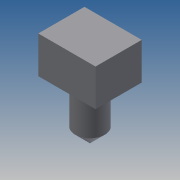
# Autodesk Inventor part: effector
Saved by Autodesk Inventor 2013 (Build 170138000, 138)
## iProperties
Created: 2017-03-06
Part Number: effector
Material: Generic
Document SubType Name: Modeling
Designer: employee
Density: 1 g/cm^3
Author: employee
Autodesk Inventor part; units mm, degrees
ref_plane "YZ Plane" through (0, 0, 0) normal (1, 0, 0) x (0, 1, 0)
ref_plane "XZ Plane" through (0, 0, 0) normal (0, 1, 0) x (-1, 0, 0)
ref_plane "XY Plane" through (0, 0, 0) normal (0, 0, 1) x (1, 0, 0)
sketch "Sketch1" plane through (0, 0, 0) normal (0, 1, 0) x (-1, 0, 0)
  line L0 (0, 0) -> (8, 8)
  line L1 (8, 8) -> (8, 50)
  line L2 (8, 50) -> (0, 50)
  line L3 (0, 50) -> (0, 0)
  dimension "d0" = 50
  dimension "d1" = 8
  dimension "d2" = 135
  constraints: 8 end point, 2 perpendicular, 1 vertical
  measures "d0" distance of L2.end L0.start
  measures "d1" distance between parallel lines of L1 L3
  measures "d2" angle of L3 L0
revolve "Revolution1" add sketch "Sketch1" angle 360 about axis through (0, 0, 50) along (0, 0, -1)
sketch "Sketch2" plane through (0, 0, 50) normal (0, 0, 1) x (1, 0, 0)
  circle A0 centre (0, 0) radius 8 projected
  line L0 (-15.5, -12.5) -> (15.5, -12.5)
  line L1 (15.5, -12.5) -> (15.5, 12.5)
  line L2 (15.5, 12.5) -> (-15.5, 12.5)
  line L3 (-15.5, 12.5) -> (-15.5, -12.5)
  line L4 (-15.5, -12.5) -> (15.5, 12.5) construction
  line L5 (15.5, -12.5) -> (-15.5, 12.5) construction
  dimension "d4" = 31
  dimension "d6" = 25
  constraints: 12 end point, 2 midpoint, 2 parallel, 1 horizontal, 1 perpendicular
  measures "d4" distance of L0.start L0.end
  measures "d6" distance of L2.end L0.start
extrude "Extrusion1" add sketch "Sketch2" against normal blind 20
body "Solid1"
